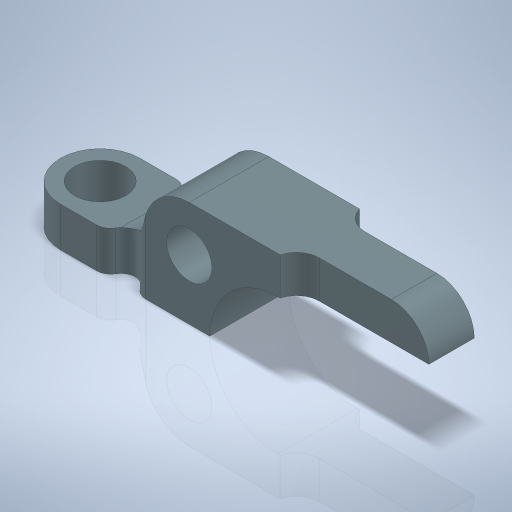
# Autodesk Inventor part: KippHebel
Saved by Autodesk Inventor 2024 (Build 280153000, 153)
## iProperties
Created: 2024-07-16
Part Number: KippHebel
Material: Blei
Document SubType Name: Modeling
Designer: ffogue
Density: 11.34 g/cm^3
Appearance: Blei
Author: ffogue
Autodesk Inventor part; units mm, degrees
note: some values were not read from the file. Chosen so that the rebuilt part matches the saved one: direction of "Bohrung1"; direction of "Bohrung2".
ref_plane "YZ Plane" through (0, 0, 0) normal (1, 0, 0) x (0, 1, 0)
ref_plane "XY Plane" through (0, 0, 0) normal (0, 0, 1) x (1, 0, 0)
sketch "Skizze1" plane through (0, 0, 0) normal (0, 1, 0) x (-1, 0, 0)
  line L0 (0, 0) -> (-16.65, 0)
  arc A0 (-16.65, 0) -> (-22.65, 6) centre (-22.65, 0) ccw
  line L1 (-22.65, 6) -> (-34.45, 6)
  arc A1 (-31.15, 9.3) -> (-34.45, 6) centre (-31.15, 6) ccw
  line L2 (-31.15, 9.3) -> (-14.85, 9.3)
  arc A2 (-10.9092, 5.9857) -> (-14.85, 9.3) centre (-14.85, 5.3) ccw
  arc A3 (-10.9092, 5.9857) -> (-7.9536, 3.5) centre (-7.9536, 6.5) ccw
  line L3 (-7.9536, 3.5) -> (0, 3.5)
  line L4 (0, 3.5) -> (0, 0)
  dimension "d0" = 3
  dimension "d1" = 4
  dimension "d2" = 3.5
  dimension "d3" = 7.8
  dimension "d4" = 3.3
  dimension "d5" = 6
  dimension "d6" = 14.85
  dimension "d7" = 19.6
  constraints: 10 end point, 8 point on circle, 5 tangent, 4 centre point, 3 parallel, 2 point on line, 1 horizontal, 1 perpendicular
  measures "d0" radius of A3
  measures "d1" radius of A2
  measures "d2" distance between parallel lines of L0 L3
  measures "d3" horizontal distance of A0.centre A2.centre
  measures "d4" distance between parallel lines of L1 L2
  measures "d5" radius of A0
  measures "d6" distance from line of L4 A2.centre
  measures "d7" horizontal distance of L1.end A2.centre
extrude "Extrusion1" add sketch "Skizze1" along normal blind 7
sketch "Skizze3" plane through (0, 0, 0) normal (0, -1, 0) x (1, 0, 0)
  arc A0 (14.85, 9.3) -> (10.9092, 5.9857) centre (14.85, 5.3) ccw projected
  point P0 (0, 0)
  constraints: 1 coincident
hole "Bohrung1" at (14.85, 0, 5.3) direction (0, 1, 0) diameter 4 depth 7
sketch "Skizze4" plane through (14.85, 0, 9.3) normal (0, 0, 1) x (1, 0, 0)
  line L0 (-2, 7) -> (2, 7) projected
  line L1 (2, 0) -> (-2, 0) projected
  line L2 (0, 0) -> (0, 7) construction
  line L3 (0, 7) -> (0, 0) construction
  line L4 (1.8, 0) -> (-14.85, 0) projected
  arc A0 (-4.75, 0) -> (-7.25, 0) centre (-6, 0) ccw
  dimension "d17" = 1.25
  dimension "d18" = 6
  constraints: 3 point on line, 2 end point, 2 point on circle, 1 centre point, 1 midpoint, 1 vertical
  measures "d17" radius of A0
  measures "d18" distance from line of L2 A0.centre
extrude "Extrusion2" cut sketch "Skizze4" against normal up to surface (9.3 mm away)
fillet "Rundung1" radius 1.25 2 edges at (10.1, 0, 2.202) (7.6, 0, 1.75)
ref_plane "Arbeitsebene1" through (0, 3.5, 0) normal (0, 1, 0) x (-1, 0, 0)
mirror "Spiegeln1" about plane through (0, 3.5, 0) normal (0, 1, 0) of "Extrusion2", "Rundung1"
fillet "Rundung2" radius 3.5 2 edges at (0, 0, 1.75) (0, 7, 1.75)
sketch "Skizze5" plane through (7.9536, 0.8712, 3.5) normal (0, 0, 1) x (1, 0, 0)
  arc A0 (-4.4536, 6.1288) -> (-4.4536, -0.8712) centre (-4.4536, 2.6288) ccw projected
  point P0 (-7.9536, -0.8712)
  constraints: 1 coincident
hole "Bohrung2" at (3.5, 3.5, 3.5) direction (0, 0, -1) diameter 4.5 depth 3.5
sketch "Skizze6" plane through (14.85, 0, 9.3) normal (0, 0, 1) x (1, 0, 0)
  line L0 (0, 0) -> (16.3, 0) projected
  line L1 (16.3, 0) -> (16.3, 7) projected
  line L2 (0, 7) -> (16.3, 7) projected
  line L3 (0, 0) -> (0, 7) projected
  line L4 (16.3, 0) -> (19.6, 0) projected
  line L5 (19.6, 0) -> (19.6, 7) projected
  line L6 (16.3, 7) -> (19.6, 7) projected
  line L7 (16.3, 0) -> (16.3, 7) projected
  line L8 (8, 5.5) -> (19.6, 5.5)
  line L9 (8, 5.5) -> (8, 7)
  point P0 (-14.85, 0)
  point P1 (8, 6.25)
  dimension "d32" = 1.5
  dimension "d38" = 8
  constraints: 4 end point, 2 perpendicular, 2 point on line, 1 midpoint
  measures "d32" distance between parallel lines of L6 L8
  measures "d38" distance from line of point (8, 6.25) L3
extrude "Extrusion5" cut sketch "Skizze6" against normal up to surface (3.3 mm away) contours L8 L9 L2 L1 | L1 L6 L5 L8
mirror "Spiegeln2" about plane through (0, 3.5, 0) normal (0, 1, 0) of "Extrusion5"
fillet "Rundung3" radius 2 2 edges at (22.85, 5.5, 7.65) (22.85, 1.5, 7.65)
